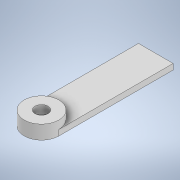
# Autodesk Inventor part: wheel_stabilizer
Saved by Autodesk Inventor 2021 (Build 250183000, 183)
## iProperties
Created: 2021-03-10
Part Number: wheel_stabilizer
Material: Generic
Document SubType Name: Modeling
Designer: Mateusz
Density: 1 g/cm^3
Appearance: Default
Author: Mateusz
Autodesk Inventor part; units mm, degrees
ref_plane "YZ Plane" through (0, 0, 0) normal (1, 0, 0) x (0, 1, 0)
ref_plane "XZ Plane" through (0, 0, 0) normal (0, 1, 0) x (-1, 0, 0)
ref_plane "XY Plane" through (0, 0, 0) normal (0, 0, 1) x (1, 0, 0)
sketch "Sketch1" plane through (0, 0, 0) normal (0, 1, 0) x (-1, 0, 0)
  circle A0 centre (0, 0) radius 11.25
  arc A1 (21.25, 0) -> (-21.25, 0) centre (0, 0) ccw
  line L0 (0, -140) -> (21.25, -140)
  line L1 (21.25, -140) -> (-21.25, -140)
  line L2 (-21.25, -140) -> (-21.25, 0)
  line L3 (21.25, -140) -> (21.25, 0)
  dimension "d0" = 22.5
  constraints: 8 end point, 2 centre point, 2 coincident, 2 point on circle, 1 perpendicular, 1 point on line, 1 tangent
  measures "d0" diameter of A0
extrude "Extrusion1" add sketch "Sketch1" along normal blind 7
sketch "Sketch2" plane through (0, 7, 0) normal (0, 1, 0) x (1, 0, 0)
  circle A0 centre (0, 0) radius 11.25 projected
  circle A1 centre (0, 0) radius 21.25
  circle A2 centre (0, 0) radius 8
  dimension "d5" = 16
  constraints: 2 centre point, 2 coincident
  measures "d5" diameter of A2
extrude "Extrusion2" add sketch "Sketch2" along normal blind 10 contours A0 | A1
sketch "Sketch3" plane through (0, 7, 0) normal (0, 1, 0) x (1, 0, 0)
  point P0 (0, 0)
body "Solid1"
